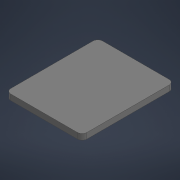
# Autodesk Inventor part: Tapa Case
Saved by Autodesk Inventor 2021 (Build 250183000, 183)
## iProperties
Created: 2021-03-29
Part Number: Tapa Case
Material: Genérico
Document SubType Name: Modeling
Designer: grego
Density: 1 g/cm^3
Appearance: Valor por defecto
Author: grego
Autodesk Inventor part; units mm, degrees
ref_plane "YZ Plane" through (0, 0, 0) normal (1, 0, 0) x (0, 1, 0)
ref_plane "XZ Plane" through (0, 0, 0) normal (0, 1, 0) x (-1, 0, 0)
ref_plane "XY Plane" through (0, 0, 0) normal (0, 0, 1) x (1, 0, 0)
sketch "Boceto1" plane through (0, 0, 0) normal (0, 1, 0) x (-1, 0, 0)
  line L0 (-5, 0) -> (-75.1, 0)
  line L1 (-80.1, -5) -> (-80.1, -91.5)
  line L2 (-75.1, -96.5) -> (-5, -96.5)
  line L3 (0, -91.5) -> (0, -5)
  arc A0 (0, -5) -> (-5, 0) centre (-5, -5) ccw
  arc A1 (-75.1, 0) -> (-80.1, -5) centre (-75.1, -5) ccw
  arc A2 (-80.1, -91.5) -> (-75.1, -96.5) centre (-75.1, -91.5) ccw
  arc A3 (-5, -96.5) -> (0, -91.5) centre (-5, -91.5) ccw
  point P0 (0, 0)
  point P1 (-80.1, -96.5)
  point P2 (-80.1, 0)
  point P3 (0, -96.5)
  dimension "d0" = 96.5
  dimension "d1" = 80.1
  dimension "d2" = 5
  constraints: 8 end point, 8 point on circle, 8 point on line, 8 tangent, 4 centre point, 3 equal radius, 2 parallel, 1 horizontal, 1 perpendicular
  measures "d0" distance of point (-80.1, 0) point (-80.1, -96.5)
  measures "d1" distance of point (-80.1, -96.5) point (0, -96.5)
  measures "d2" radius of A0
extrude "Extrusión1" add sketch "Boceto1" along normal blind 6
